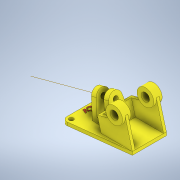
# Autodesk Inventor part: Ricea f. Florentina alexandra-T1
Saved by Autodesk Inventor 2022 (Build 260153000, 153)
## iProperties
Created: 2022-02-18
Part Number: Ricea f. Florentina alexandra-T1
Material: Steel, Carbon
Document SubType Name: Modeling
Designer: mtrot
Density: 7.85 g/cm^3
Appearance: Canary
Student_ACE: Ricea f. Florentina alexandra
Grupa_ACE: CR-3
Tema_ACE: 1-Reper parametric
An_ACE: 2022
Author: mtrot
Autodesk Inventor part; units mm, degrees
ref_plane "YZ Plane" through (0, 0, 0) normal (1, 0, 0) x (0, 1, 0)
ref_plane "XZ Plane" through (0, 0, 0) normal (0, 1, 0) x (-1, 0, 0)
ref_plane "XY Plane" through (0, 0, 0) normal (0, 0, 1) x (1, 0, 0)
sketch "Sketch1" plane through (0, 0, 0) normal (0, 0, 1) x (1, 0, 0)
  line L0 (-28.9877, 0) -> (173.9264, 0) projected
  line L1 (-29.4372, -7.8877) -> (176.6233, 47.3261) projected
  line L2 (101.2142, 39.5436) -> (109.9075, 41.8729)
  line L3 (109.9075, 41.8729) -> (118.9662, 8.0655)
  line L4 (118.9662, 8.0655) -> (132.4891, 11.689)
  line L5 (132.4891, 11.689) -> (123.4305, 45.4964)
  line L6 (123.4305, 45.4964) -> (132.1238, 47.8258)
  line L7 (132.1238, 47.8258) -> (144.9387, 0)
  line L8 (144.9387, 0) -> (111.8098, 0)
  line L9 (111.8098, 0) -> (101.2142, 39.5436)
  point P0 (0, 0)
  dimension "d0" = 12
  dimension "d1" = 9
  dimension "d2" = 14
  dimension "d3" = 9
  dimension "d4" = 117
  dimension "d5" = 35
  constraints: 16 end point, 3 perpendicular, 2 parallel, 2 point on line, 1 collinear, 1 horizontal
  measures "d0" distance between parallel lines of L6 L1
  measures "d1" distance of L2.start L2.end
  measures "d2" distance between parallel lines of L5 L3
  measures "d3" distance of L5.end L6.end
  measures "d4" distance from line of L3 point (0, 0)
  measures "d5" distance between parallel lines of L4 L2
extrude "Extrusion1" add sketch "Sketch1" along normal mid plane 50 contours L9 L1 L3 L4 L5 L7 L0 | L9 L2 L3 L1 | L1 L5 L6 L7
sketch "Sketch2" plane through (111.8098, 0, -25) normal (-0.9659258, -0.258819, 0) x (0, 0, 1)
  line L0 (0, 40.9385) -> (50, 40.9385) projected
  line L1 (25, 64.8401) -> (25, -46.4712) projected
  line L2 (0, -8.5744) -> (50, -8.5744) projected
  line L3 (1.57, -23.5744) -> (48.43, -23.5744)
  arc A0 (36.7378, 31.4335) -> (13.2622, 31.4335) centre (25, 28.9385) ccw
  line L4 (48.43, -23.5744) -> (36.7378, 31.4335)
  line L5 (1.57, -23.5744) -> (13.2622, 31.4335)
  point P0 (25, 28.9385)
  dimension "d8" = 15
  dimension "d9" = 78
  dimension "d10" = 78
  dimension "d11" = 12
  constraints: 6 end point, 3 tangent, 2 point on circle, 1 centre point, 1 horizontal, 1 point on line
  measures "d8" distance between parallel lines of L3 L2
  measures "d9" angle of L3 L5
  measures "d10" angle of L3 L4
  measures "d11" radius of A0
extrude "Extrusion2" cut sketch "Sketch2" against normal through all keep common part
sketch "Sketch3" plane through (0, 0, 0) normal (0, 0, 1) x (1, 0, 0)
  line L0 (139.7623, 0) -> (132.9832, 25.3)
  line L1 (132.9832, 25.3) -> (156.1654, 31.5117)
  line L2 (156.1654, 31.5117) -> (153.5822, 41.1522)
  line L3 (153.5822, 41.1522) -> (182.56, 48.9168)
  line L4 (182.56, 48.9168) -> (195.6672, 0)
  line L5 (195.6672, 0) -> (139.7623, 0)
  line L6 (-40.5532, -10.8662) -> (234.4172, 62.8119) projected
  line L7 (-38.7334, 0) -> (232.4003, 0) projected
  line L8 (134.5839, 38.6446) -> (144.9387, 0) projected
  point P0 (0, 0)
  dimension "d14" = 5
  dimension "d15" = 25.3
  dimension "d16" = 49
  dimension "d17" = 30
  constraints: 12 end point, 4 perpendicular, 2 collinear, 1 horizontal
  measures "d14" distance between parallel lines of L8 L0
  measures "d15" vertical distance of L0.start L0.end
  measures "d16" distance between parallel lines of L4 L8
  measures "d17" distance between parallel lines of L2 L4
extrude "Extrusion3" add sketch "Sketch3" along normal mid plane 61 contours L0 L1 L8 L5 | L8 L1 L2 L3 L4 L5
sketch "Sketch4" plane through (153.5822, 41.1522, 30.5) normal (-0.258819, 0.9659258, 0) x (0.9659258, 0.258819, 0)
  line L0 (35, 56) -> (-19, 56)
  line L1 (-19, 56) -> (-19, 5)
  line L2 (-19, 5) -> (35, 5)
  line L3 (35, 5) -> (35, 56)
  line L4 (30, 61) -> (30, 0) projected
  line L5 (30, 0) -> (0, 0) projected
  line L6 (-24, 61) -> (0, 61) projected
  line L7 (-24, 16.1105) -> (-24, 0) projected
  point P0 (-159, 30.5)
  dimension "d20" = 5
  dimension "d21" = 5
  dimension "d22" = 5
  dimension "d23" = 5
  constraints: 8 end point, 2 parallel, 1 horizontal, 1 perpendicular
  measures "d20" distance between parallel lines of L4 L3
  measures "d21" distance between parallel lines of L5 L2
  measures "d22" distance between parallel lines of L6 L0
  measures "d23" distance between parallel lines of L7 L1
extrude "Extrusion4" cut sketch "Sketch4" against normal through all
sketch "Sketch5" plane through (0, 0, 0) normal (0, 0, 1) x (1, 0, 0)
  circle A0 centre (168.0711, 45.0345) radius 15
  line L0 (182.56, 48.9168) -> (195.6672, 0) projected
  line L1 (153.5822, 41.1522) -> (182.56, 48.9168) projected
  point P0 (0, 0)
  dimension "d26" = 30
  constraints: 1 centre point, 1 midpoint, 1 tangent
  measures "d26" diameter of A0
extrude "Extrusion5" add sketch "Sketch5" along normal mid plane 71
sketch "Sketch6" plane through (0, 0, 0) normal (0, 0, 1) x (1, 0, 0)
  circle A0 centre (168.0711, 45.0345) radius 19.5
  circle A1 centre (168.0711, 45.0345) radius 15 projected
  point P0 (0, 0)
  dimension "d29" = 39
  constraints: 1 centre point, 1 concentric
  measures "d29" diameter of A0
extrude "Extrusion6" cut sketch "Sketch6" along normal mid plane 41 contours A0 | A1
sketch "Sketch7" plane through (0, 0, 0) normal (0, 1, 0) x (-1, 0, 0)
  line L0 (-234.8006, 0) -> (39.1334, 0) projected
  line L1 (-91.6172, 42.9434) -> (-195.6672, 30.5)
  line L2 (-195.6672, 30.5) -> (-195.6672, -30.5)
  line L3 (-195.6672, -30.5) -> (-91.6172, -42.9434)
  line L4 (-82.6672, -35) -> (-82.6672, 35)
  arc A0 (-91.6172, -42.9434) -> (-82.6672, -35) centre (-90.6672, -35) ccw
  arc A1 (-82.6672, 35) -> (-91.6172, 42.9434) centre (-90.6672, 35) ccw
  point P0 (0, 0)
  dimension "d32" = 8
  dimension "d33" = 8
  dimension "d34" = 113
  dimension "d35" = 70
  dimension "d36" = 35
  constraints: 8 end point, 4 point on circle, 4 tangent, 2 centre point, 2 coincident, 1 vertical
  measures "d32" radius of A0
  measures "d33" radius of A1
  measures "d34" distance between parallel lines of L4 L2
  measures "d35" distance of A1.centre A0.centre
  measures "d36" distance from line of A0.centre L0
extrude "Extrusion7" add sketch "Sketch7" against normal blind 6
sketch "Sketch8" plane through (168.0711, 45.0345, 35.5) normal (0, 0, 1) x (1, 0, 0)
  circle A0 centre (0, 0) radius 15 projected
  point P0 (-168.0711, -45.0345)
  constraints: 1 coincident
hole "Hole1" at (168.0711, 45.0345, 35.5) direction (0, 0, -1) diameter 15 end through all
sketch "Sketch9" plane through (0, 0, 0) normal (0, 1, 0) x (1, 0, 0)
  arc A0 (91.6172, 42.9434) -> (82.6672, 35) centre (90.6672, 35) ccw projected
  point P0 (0, 0)
  constraints: 1 coincident
hole "Hole2" at (90.6672, 0, -35) direction (0, -1, 0) diameter 8 end through all
sketch "Sketch10" plane through (0, 0, 0) normal (0, 1, 0) x (1, 0, 0)
  arc A0 (82.6672, -35) -> (91.6172, -42.9434) centre (90.6672, -35) ccw projected
  point P0 (0, 0)
  constraints: 1 coincident
hole "Hole3" at (90.6672, 0, 35) direction (0, -1, 0) diameter 8 end through all
sketch "Sketch11" plane through (104.32, 27.9525, 0) normal (-0.9659258, -0.258819, 0) x (0, 0, 1)
  arc A0 (11.7378, 2.4949) -> (-11.7378, 2.4949) centre (0, 0) ccw projected
  point P0 (0, 0)
  constraints: 1 coincident
hole "Hole4" at (104.32, 27.9525, 0) direction (0.9659258, 0.258819, 0) diameter 9 end through all
sketch "Sketch12" plane through (0, 0, 0) normal (0, 1, 0) x (1, 0, 0)
  line L0 (97.6672, 14.5) -> (97.6672, -14.5) construction
  line L1 (97.6672, -14.5) -> (86.6672, -14.5) construction
  line L2 (86.6672, -14.5) -> (86.6672, 14.5) construction
  line L3 (86.6672, 14.5) -> (97.6672, 14.5) construction
  line L4 (82.6672, 35) -> (82.6672, -35) projected
  spline S0 degree 2 poles (86.9646, 8.5697) (86.9646, 10.5875) (88.9095, 12.7593) (90.7896, 12.7593) knots 0 0 0 1 2 2 2
  line L5 (90.7896, 12.7593) -> (97.1753, 12.7593)
  line L6 (97.1753, 12.7593) -> (97.1753, 10.2472)
  line L7 (97.1753, 10.2472) -> (90.9354, 10.2472)
  spline S1 degree 2 poles (90.9354, 10.2472) (89.8901, 10.2472) (88.869, 9.4611) (88.869, 8.5697) knots 0 0 0 1 2 2 2
  spline S2 degree 2 poles (88.869, 8.5697) (88.869, 7.7026) (89.8495, 6.8922) (90.9354, 6.8922) knots 0 0 0 1 2 2 2
  line L8 (90.9354, 6.8922) -> (97.1753, 6.8922)
  line L9 (97.1753, 6.8922) -> (97.1753, 4.3801)
  line L10 (97.1753, 4.3801) -> (90.7977, 4.3801)
  spline S3 degree 2 poles (90.7977, 4.3801) (88.95, 4.3801) (86.9646, 6.4951) (86.9646, 8.5697) knots 0 0 0 1 2 2 2
  spline S4 degree 2 poles (86.9808, -1.8598) (86.9808, 0.393) (89.7037, 3.0348) (92.1672, 3.0348) knots 0 0 0 1 2 2 2
  spline S5 degree 2 poles (92.1672, 3.0348) (94.5416, 3.0348) (97.3698, 0.3849) (97.3698, -1.8679) knots 0 0 0 1 2 2 2
  spline S6 degree 2 poles (97.3698, -1.8679) (97.3698, -2.4595) (97.232, -3.4157) (97.1186, -3.8533) knots 0 0 0 1 2 2 2
  spline S7 degree 2 poles (97.1186, -3.8533) (97.0132, -4.1937) (96.6648, -4.9959) (96.5351, -5.2472) knots 0 0 0 1 2 2 2
  line L11 (96.5351, -5.2472) -> (94.1526, -5.2472)
  line L12 (94.1526, -5.2472) -> (94.1526, -4.9959)
  spline S8 degree 2 poles (94.1526, -4.9959) (94.3147, -4.8096) (94.7685, -4.2585) (94.9792, -3.91) knots 0 0 0 1 2 2 2
  spline S9 degree 2 poles (94.9792, -3.91) (95.198, -3.5616) (95.4978, -2.7269) (95.4978, -2.265) knots 0 0 0 1 2 2 2
  spline S10 degree 2 poles (95.4978, -2.265) (95.4978, -1.722) (95.1575, -0.8225) (94.728, -0.4092) knots 0 0 0 1 2 2 2
  spline S11 degree 2 poles (94.728, -0.4092) (94.3471, -0.0365) (93.0424, 0.4417) (92.1591, 0.4417) knots 0 0 0 1 2 2 2
  spline S12 degree 2 poles (92.1591, 0.4417) (91.2272, 0.4417) (89.9549, -0.0527) (89.5659, -0.4579) knots 0 0 0 1 2 2 2
  spline S13 degree 2 poles (89.5659, -0.4579) (89.185, -0.8468) (88.8528, -1.8031) (88.8528, -2.2812) knots 0 0 0 1 2 2 2
  spline S14 degree 2 poles (88.8528, -2.2812) (88.8528, -2.7755) (89.185, -3.675) (89.3876, -3.983) knots 0 0 0 1 2 2 2
  spline S15 degree 2 poles (89.3876, -3.983) (89.5902, -4.3233) (90.0197, -4.8339) (90.1899, -5.0203) knots 0 0 0 1 2 2 2
  line L13 (90.1899, -5.0203) -> (90.1899, -5.2472)
  line L14 (90.1899, -5.2472) -> (87.8398, -5.2472)
  spline S16 degree 2 poles (87.8398, -5.2472) (87.7101, -4.9716) (87.386, -4.2504) (87.2725, -3.8614) knots 0 0 0 1 2 2 2
  spline S17 degree 2 poles (87.2725, -3.8614) (87.1267, -3.3914) (86.9808, -2.5729) (86.9808, -1.8598) knots 0 0 0 1 2 2 2
  line L15 (94.7199, -13.6507) -> (87.1753, -10.9441)
  line L16 (87.1753, -10.9441) -> (87.1753, -8.3752)
  line L17 (87.1753, -8.3752) -> (94.7199, -5.6929)
  line L18 (94.7199, -5.6929) -> (94.7199, -8.1645)
  line L19 (94.7199, -8.1645) -> (89.7361, -9.7042)
  line L20 (89.7361, -9.7042) -> (94.7199, -11.2277)
  line L21 (94.7199, -11.2277) -> (94.7199, -13.6507)
  point P0 (0, 0)
  point P1 (82.6672, 0)
  point P2 (86.6672, 0)
  dimension "d67" = 15
  dimension "d68" = 29
  dimension "d69" = 11
  constraints: 2 midpoint, 1 horizontal alignment, 1 parallel, 2 other
  measures "d67" distance between parallel lines of L4 L0
  measures "d68" distance between parallel lines of L1 L3
  measures "d69" distance between parallel lines of L2 L0
emboss "Emboss1" sketch "Sketch12" operation add depth 1 direction (0, -1, 0)
equation "\"d26\" = d17"
equation "\"d29\" = 1.3 * d17"
equation "\"d36\" = 0.5 * d35"
body "Solid1"
